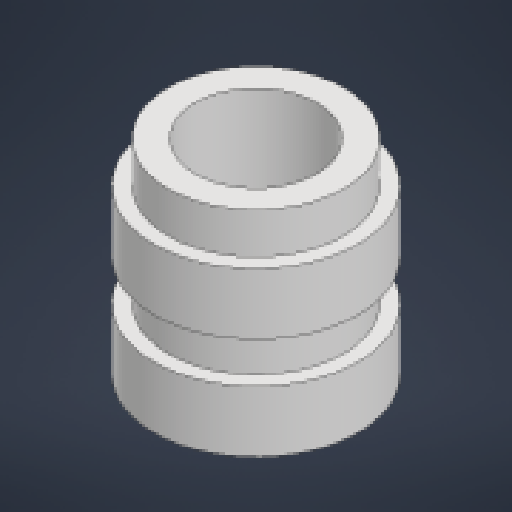
# Autodesk Inventor part: M3 heat set insert
Saved by Autodesk Inventor 2026.1 (Build 301233020, 233B)
## iProperties
Created: 2025-09-22
Part Number: M3 heat set insert
Material: Generic
Document SubType Name: Modeling
Designer: gavin
Density: 1 g/cm^3
Appearance: Default
Author: gavin
Autodesk Inventor part; units mm, degrees
ref_plane "YZ Plane" through (0, 0, 0) normal (1, 0, 0) x (0, 1, 0)
ref_plane "XZ Plane" through (0, 0, 0) normal (0, 1, 0) x (-1, 0, 0)
ref_plane "XY Plane" through (0, 0, 0) normal (0, 0, 1) x (1, 0, 0)
sketch "Sketch1" plane through (0, 0, 0) normal (1, 0, 0) x (0, 1, 0)
  line L0 (0, 0) -> (0, -2.5)
  line L1 (0, -2.5) -> (1.5, -2.5)
  line L2 (1.5, -2.5) -> (1.5, -2.15)
  line L3 (1.5, -2.15) -> (2.5, -2.15)
  line L4 (2.5, -2.15) -> (2.5, -2.5)
  line L5 (2.5, -2.5) -> (4, -2.5)
  line L6 (4, -2.5) -> (4, -2.15)
  line L7 (4, -2.15) -> (5, -2.15)
  line L8 (5, -2.15) -> (5, 0)
  line L9 (5, 0) -> (0, 0)
  line L10 (5, -1.5) -> (0, -1.5)
  point P0 (4.5, -2.15)
  dimension "d1" = 2.15
  dimension "d2" = 1.5
  dimension "d3" = 2.5
  dimension "d8" = 5
  dimension "d9" = 1.5
  dimension "d10" = 1
  dimension "d11" = 1.5
  constraints: 22 end point, 8 perpendicular, 5 point on line, 1 horizontal, 1 midpoint, 1 vertical
  measures "d1" distance between parallel lines of L9 L7
  measures "d2" distance between parallel lines of L9 L10
  measures "d3" distance between parallel lines of L9 L1
  measures "d8" distance of L8.end L0.start
  measures "d9" distance of L0.end L1.end
  measures "d10" distance of L2.end L3.end
  measures "d11" distance of L4.end L5.end
revolve "Revolution1" add sketch "Sketch1" angle 360 about axis through (0, 5, 0) along (0, -1, 0) contours L10 L8 L7 L6 L5 L4 L3 L2 L1 L0
equation "\"d11\" = d9"
body "Solid1"
